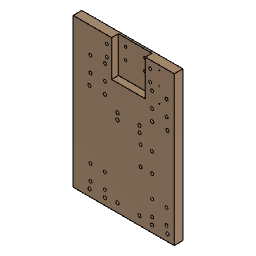
Z main board (Autodesk Fusion 360 design; units mm, degrees)
Autodesk Fusion 360 part; units mm, degrees
sketch "Z main board" plane through (0, 0, 0) normal (0, 1, 0) x (1, 0, 0)
  circle A0 centre (89, -64) radius 3
  circle A1 centre (33, -7.5) radius 3.25
  circle A2 centre (-10, -109.5) radius 2.5
  line L0 (-71, -60) -> (-71, 150) construction
  line L1 (-80, -64) -> (100, -64) construction
  circle A3 centre (-71, -40.5) radius 3.25
  circle A4 centre (30, -133.4799) radius 2.5
  line L2 (45, -74.5) -> (-25, -74.5)
  line L3 (-70, -109.5) -> (80, -109.5) construction
  line L4 (45, -149.5) -> (45, -74.5)
  line L5 (-70, -133.5) -> (80, -133.5) construction
  line L6 (30, -133.4799) -> (30, -109.5) construction
  circle A5 centre (-35, -133.4853) radius 3
  circle A6 centre (55, -133.5) radius 3
  circle A7 centre (-35, -109.5) radius 3
  line L7 (91, -60) -> (91, 150) construction
  line L8 (-105, -149.5) -> (105, -149.5)
  line L9 (-80, -40.5) -> (100, -40.5) construction
  circle A8 centre (-69, -64) radius 3
  circle A9 centre (-13, -20.5) radius 3.25
  circle A10 centre (91, -40.5) radius 3.25
  line L10 (-20, -20.5) -> (45, -20.5) construction
  circle A11 centre (89, -96) radius 3
  line L11 (-13, -80) -> (-13, 145.5) construction
  line L12 (-105, 159.5) -> (-105, -149.5)
  circle A12 centre (-13, -7.5) radius 3.25
  line L13 (-69, -140) -> (-69, 140) construction
  line L14 (-39, -130) -> (-39, 150) construction
  circle A13 centre (-39, -96) radius 3
  circle A14 centre (-39, -64) radius 3
  circle A15 centre (30, -109.5) radius 2.5
  line L15 (59, -130) -> (59, 150) construction
  circle A16 centre (89, 99) radius 3
  line L16 (30, 13) -> (65, 13) construction
  line L17 (33, -80) -> (33, 145.5) construction
  circle A17 centre (59, 131) radius 3
  line L18 (89, 140) -> (89, -140) construction
  line L19 (35, -5) -> (35, 60) construction
  circle A18 centre (59, 53) radius 3
  line L20 (-80, 131) -> (100, 131) construction
  circle A19 centre (-69, 99) radius 3
  circle A20 centre (89, 131) radius 3
  line L21 (105, -149.5) -> (105, 159.5)
  circle A21 centre (59, 13) radius 3
  circle A22 centre (59, 145.5) radius 3.25
  circle A23 centre (35, 13) radius 3
  line L22 (105, 159.5) -> (-105, 159.5)
  line L23 (-80, 99) -> (100, 99) construction
  circle A24 centre (91, 145.5) radius 3.25
  circle A25 centre (-39, 145.5) radius 3.25
  circle A26 centre (-39, 99) radius 3
  circle A27 centre (33, 141.5) radius 3.25
  line L24 (30, 53) -> (65, 53) construction
  line L25 (-80, 145.5) -> (100, 145.5) construction
  circle A28 centre (-71, 145.5) radius 3.25
  line L26 (-20, 141.5) -> (40, 141.5) construction
  circle A29 centre (-69, 131) radius 3
  circle A30 centre (-39, 131) radius 3
  circle A31 centre (59, 99) radius 3
  circle A32 centre (35, 53) radius 3
  circle A33 centre (-13, 141.5) radius 3.25
  circle A34 centre (59, -64) radius 3
  circle A35 centre (59, -96) radius 3
  circle A36 centre (-39, -40.5) radius 3.25
  line L27 (-20, -7.5) -> (45, -7.5) construction
  line L28 (-80, -96) -> (100, -96) construction
  circle A37 centre (33, -20.5) radius 3.25
  line L29 (-25, -74.5) -> (-25, -149.5)
  line L30 (-10, -133.485) -> (-10, -109.5) construction
  line L31 (55, -134.9971) -> (55, -109.5) construction
  circle A38 centre (-10, -133.485) radius 2.5
  circle A39 centre (-69, -96) radius 3
  line L32 (-35, -133.4853) -> (-35, -109.5) construction
  circle A40 centre (59, -40.5) radius 3.25
  circle A41 centre (55, -109.5) radius 3
  line L33 (74, -32.219) -> (74, -146.1103) construction
  circle A42 centre (74, -80) radius 1
  circle A43 centre (74, -112) radius 1
  circle A44 centre (74, -140) radius 1
  dimension "d1" = 75
  dimension "d2" = 70
  dimension "d3" = 60
  dimension "d4" = 16
  dimension "d5" = 24
  dimension "d6" = 40
  dimension "d7" = 25
  dimension "d8" = 50
  dimension "d9" = 16
  dimension "d10" = 30
  dimension "d11" = 30
  dimension "d12" = 36
  dimension "d13" = 210
  dimension "d14" = 309
  dimension "d15" = 32
  dimension "d16" = 53.5
  dimension "d17" = 32
  dimension "d18" = 163
  dimension "d19" = 2
  dimension "d20" = 2
  dimension "d21" = 14.5
  dimension "d22" = 46
  dimension "d23" = 3
  dimension "d24" = 3
  dimension "d25" = 24
  dimension "d26" = 40
  dimension "d27" = 13
  dimension "d28" = 149
  dimension "d29" = 25
  dimension "d30" = 6
  dimension "d31" = 5
  dimension "d32" = 5
  dimension "d33" = 6
  dimension "d34" = 6
  dimension "d35" = 5
  dimension "d36" = 5
  dimension "d37" = 6
  dimension "d38" = 6
  dimension "d39" = 6
  dimension "d40" = 6
  dimension "d41" = 6
  dimension "d42" = 6
  dimension "d43" = 6
  dimension "d44" = 6
  dimension "d45" = 6
  dimension "d46" = 6
  dimension "d47" = 6
  dimension "d48" = 6
  dimension "d49" = 6
  dimension "d50" = 6
  dimension "d51" = 6
  dimension "d52" = 6
  dimension "d53" = 6
  dimension "d54" = 6.5
  dimension "d55" = 6.5
  dimension "d56" = 6.5
  dimension "d57" = 6.5
  dimension "d58" = 23.5
  dimension "d59" = 6.5
  dimension "d60" = 6.5
  dimension "d61" = 6.5
  dimension "d62" = 6.5
  dimension "d63" = 6.5
  dimension "d64" = 6.5
  dimension "d65" = 6.5
  dimension "d66" = 6.5
  dimension "d67" = 20
  dimension "d68" = 6.5
  dimension "d69" = 6.5
  dimension "d70" = 6
  dimension "d71" = 6
  dimension "d72" = 6
  dimension "d73" = 6
  dimension "d82" = 77
  dimension "d83" = 149
  dimension "d84" = 46
  dimension "d85" = 118
  dimension "d86" = 30
  dimension "d87" = 15
  dimension "d88" = 2
  dimension "d89" = 2
  dimension "d90" = 2
  dimension "d91" = 28
  dimension "d92" = 32
  dimension "d93" = 16
  constraint horizontal L8
  constraint perpendicular L8 L21
  constraint perpendicular L21 L22
  constraint perpendicular L8 L12
  constraint vertical L4
  constraint coincident L4.start L8
  constraint perpendicular L2 L4
  constraint coincident L29.end L8
  constraint perpendicular L8 L29
  constraint perpendicular L4 L5
  constraint perpendicular L3 L4
  constraint coincident A7.centre L3
  constraint perpendicular L3 L32
  constraint coincident A2.centre L3
  constraint perpendicular L3 L30
  constraint coincident L6.end L3
  constraint perpendicular L3 L6
  constraint coincident L31.end L3
  constraint perpendicular L3 L31
  constraint vertical L18
  constraint perpendicular L5 L15
  constraint parallel L12 L13
  constraint perpendicular L5 L14
  constraint perpendicular L18 L28
  constraint perpendicular L1 L18
  constraint perpendicular L18 L23
  constraint perpendicular L18 L20
  constraint perpendicular L0 L20
  constraint perpendicular L7 L20
  constraint perpendicular L7 L25
  constraint coincident L17.end L25
  constraint perpendicular L17 L25
  constraint perpendicular L11 L20
  constraint vertical L19
  constraint perpendicular L7 L9
  constraint perpendicular L10 L17
  constraint perpendicular L19 L27
  constraint perpendicular L15 L16
  constraint perpendicular L15 L24
  constraint perpendicular L17 L26
  constraint coincident A5.centre L32.start
  constraint coincident L30.start A38.centre
  constraint coincident A4.centre L6.start
  constraint coincident A6.centre L5
  constraint coincident A6.centre L31
  constraint coincident A7.centre L32.end
  constraint coincident A2.centre L30.end
  constraint coincident L6.end A15.centre
  constraint coincident L31.end A41.centre
  constraint coincident A13.centre L14
  constraint coincident A13.centre L28
  constraint coincident A39.centre L13
  constraint coincident A39.centre L28
  constraint coincident A8.centre L13
  constraint coincident A8.centre L1
  constraint coincident A14.centre L14
  constraint coincident A14.centre L1
  constraint coincident A35.centre L15
  constraint coincident A35.centre L28
  constraint coincident A11.centre L18
  constraint coincident A11.centre L28
  constraint coincident A34.centre L15
  constraint coincident A34.centre L1
  constraint coincident A0.centre L18
  constraint coincident A0.centre L1
  constraint coincident A31.centre L15
  constraint coincident A31.centre L23
  constraint coincident A16.centre L18
  constraint coincident A16.centre L23
  constraint coincident A17.centre L15
  constraint coincident A17.centre L20
  constraint coincident A20.centre L18
  constraint coincident A20.centre L20
  constraint coincident A26.centre L14
  constraint coincident A26.centre L23
  constraint coincident A19.centre L13
  constraint coincident A19.centre L23
  constraint coincident A29.centre L13
  constraint coincident A29.centre L20
  constraint coincident A30.centre L14
  constraint coincident A30.centre L20
  constraint coincident A25.centre L14
  constraint coincident A25.centre L25
  constraint coincident A22.centre L15
  constraint coincident A22.centre L25
  constraint coincident A24.centre L25
  constraint coincident A24.centre L7
  constraint coincident A28.centre L0
  constraint coincident A28.centre L25
  constraint coincident A3.centre L0
  constraint coincident A3.centre L9
  constraint coincident A36.centre L9
  constraint coincident A36.centre L14
  constraint coincident A40.centre L9
  constraint coincident A40.centre L15
  constraint coincident A10.centre L7
  constraint coincident A10.centre L9
  constraint coincident A9.centre L11
  constraint coincident A9.centre L10
  constraint coincident A37.centre L17
  constraint coincident A37.centre L10
  constraint coincident A12.centre L11
  constraint coincident A12.centre L27
  constraint coincident A1.centre L17
  constraint coincident A1.centre L27
  constraint coincident A33.centre L11
  constraint coincident A33.centre L26
  constraint coincident A27.centre L17
  constraint coincident A27.centre L26
  constraint coincident A23.centre L19
  constraint coincident A23.centre L16
  constraint coincident A21.centre L15
  constraint coincident A21.centre L16
  constraint coincident A18.centre L15
  constraint coincident A18.centre L24
  constraint coincident A32.centre L19
  constraint coincident A32.centre L24
  constraint perpendicular L28 L33
  constraint coincident L33 A42.centre
  constraint coincident L33 A43.centre
  constraint coincident L33 A44.centre
  measures "d1" distance of L4.start L2.start
  measures "d2" distance of L2.end L2.start
  measures "d3" distance of L4 L21
  measures "d4" distance of L5 L8
  measures "d5" distance of L3 L5
  measures "d6" distance of L30.start A4.centre
  measures "d7" distance of A5.centre L30.start
  measures "d8" distance of L31.start L21
  measures "d9" distance of L18 L21
  measures "d10" distance of L15 L18
  measures "d11" distance of L13 L14
  measures "d12" distance of L12 L13
  measures "d13" distance of L12 L21
  measures "d14" distance of L8 L22
  measures "d15" distance of L1 L28
  measures "d16" distance of L8 L28
  measures "d17" distance of L20 L23
  measures "d18" distance of L1 L23
  measures "d19" distance of L0 L13
  measures "d20" distance of L7 L18
  measures "d21" distance of L20 L25
  measures "d22" distance of L11 L17
  measures "d23" distance of L6 L17
  measures "d24" distance of L11 L30
  measures "d25" distance of L15 L19
  measures "d26" distance of L16 L24
  measures "d27" distance of L10 L27
  measures "d28" distance of L26 L27
  measures "d29" distance of L6 L31
  measures "d30" diameter of A5
  measures "d31" diameter of A38
  measures "d32" diameter of A4
  measures "d33" diameter of A6
  measures "d34" diameter of A7
  measures "d35" diameter of A2
  measures "d36" diameter of A15
  measures "d37" diameter of A41
  measures "d38" diameter of A13
  measures "d39" diameter of A39
  measures "d40" diameter of A8
  measures "d41" diameter of A14
  measures "d42" diameter of A35
  measures "d43" diameter of A11
  measures "d44" diameter of A34
  measures "d45" diameter of A0
  measures "d46" diameter of A31
  measures "d47" diameter of A16
  measures "d48" diameter of A17
  measures "d49" diameter of A20
  measures "d50" diameter of A26
  measures "d51" diameter of A19
  measures "d52" diameter of A29
  measures "d53" diameter of A30
  measures "d54" diameter of A25
  measures "d55" diameter of A22
  measures "d56" diameter of A24
  measures "d57" diameter of A28
  measures "d58" distance of L1 L9
  measures "d59" diameter of A3
  measures "d60" diameter of A36
  measures "d61" diameter of A40
  measures "d62" diameter of A10
  measures "d63" diameter of A9
  measures "d64" diameter of A37
  measures "d65" diameter of A12
  measures "d66" diameter of A1
  measures "d67" distance of L9 L10
  measures "d68" diameter of A33
  measures "d69" diameter of A27
  measures "d70" diameter of A23
  measures "d71" diameter of A21
  measures "d72" diameter of A18
  measures "d73" diameter of A32
  measures "d82" distance of A34.centre A21.centre
  measures "d83" distance of A35.centre A18.centre
  measures "d84" distance of A31.centre A18.centre
  measures "d85" distance of A17.centre A21.centre
  measures "d86" distance of A34.centre A0.centre
  measures "d87" distance of L18 L33
  measures "d88" diameter of A42
  measures "d89" diameter of A43
  measures "d90" diameter of A44
  measures "d91" distance of A43.centre A44.centre
  measures "d92" distance of A42.centre A43.centre
  measures "d93" distance of L1 A42.centre
extrude "Extrude2" add sketch "Z main board" against normal blind 10 contours L2 L4 L8 L12 L21 L22 L29
extrude "Extrude3" add sketch "Z main board" against normal blind 4 contours L2 L4 L8 L29
extrude "Extrude4" add 1 faces at (-52.0966, -10, -17.5607) along direction (0, -1, 0) blind 8
equation "d87 = 30.0 mm / 2"
equation "d89 = d88"
equation "d90 = d88"
equation "d93 = d15 / 2"
named bodies: "Z main board"
